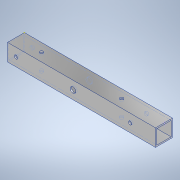
# Autodesk Inventor part: ロボットベース15x15_3
Saved by Autodesk Inventor 2020.3 (Build 243373000, 373)
## iProperties
Created: 2020-07-04
Part Number: ロボットベース15x15_3
Material: アルミニウム 6061
Document SubType Name: Modeling
Designer: totot
Density: 2.7 g/cm^3
Appearance: アルミニウム - フラット
Mass: 20.4359 g
Surface Area: 128.754 cm^2
Volume: 7.56886 cm^3
Author: totot
Autodesk Inventor part; units mm, degrees
ref_plane "YZ Plane" through (0, 0, 0) normal (1, 0, 0) x (0, 1, 0)
ref_plane "XZ Plane" through (0, 0, 0) normal (0, 1, 0) x (-1, 0, 0)
ref_plane "XY Plane" through (0, 0, 0) normal (0, 0, 1) x (1, 0, 0)
sketch "スケッチ1" plane through (0, 0, 0) normal (1, 0, 0) x (0, 1, 0)
  line L0 (0, 0) -> (-15, 0)
  line L1 (-15, 0) -> (-15, 15)
  line L2 (-15, 15) -> (0, 15)
  line L3 (0, 15) -> (0, 0)
  line L4 (-1.2, 13.8) -> (-13.8, 13.8)
  line L5 (-13.8, 13.8) -> (-13.8, 1.2)
  line L6 (-13.8, 1.2) -> (-1.2, 1.2)
  line L7 (-1.2, 1.2) -> (-1.2, 13.8)
  dimension "d0" = 15
  dimension "d1" = 15
  dimension "d2" = 1.2
  dimension "d3" = 1.2
  dimension "d4" = 1.2
  dimension "d5" = 1.2
  constraints: 16 end point, 4 parallel, 2 horizontal, 2 perpendicular
  measures "d0" distance of L1.end L2.end
  measures "d1" distance of L0.end L1.end
  measures "d2" distance between parallel lines of L2 L4
  measures "d3" distance between parallel lines of L7 L3
  measures "d4" distance between parallel lines of L1 L5
  measures "d5" distance between parallel lines of L0 L6
extrude "押し出し1" add sketch "スケッチ1" along normal blind 116
sketch "スケッチ2" plane through (0, -15, 15) normal (0, 0, 1) x (1, 0, 0)
  line L0 (0, 15) -> (116, 15) projected
  line L1 (0, 15) -> (0, 0) projected
  line L2 (116, 15) -> (116, 0) projected
  point P0 (7.5, 7.5)
  point P1 (108.5, 7.5)
  dimension "d8" = 7.5
  dimension "d9" = 7.5
  dimension "d10" = 7.5
  dimension "d11" = 7.5
  measures "d8" distance from line of L0 point (7.5, 7.5)
  measures "d9" distance from line of point (108.5, 7.5) L0
  measures "d10" distance from line of point (7.5, 7.5) L1
  measures "d11" distance from line of point (108.5, 7.5) L2
hole "穴1" at (7.5, -7.5, 15) at (108.5, -7.5, 15) direction (0, 0, -1) diameter 3 end through all
sketch "スケッチ3" plane through (0, -15, 0) normal (0, 0, -1) x (-1, 0, 0)
  circle A0 centre (-7.5, 7.5) radius 1.5 projected
  line L0 (0, 0) -> (-116, 0) projected
  point P0 (0, 15)
  point P1 (-58, 7.5)
  dimension "d19" = 50.5
  dimension "d20" = 7.5
  measures "d19" distance of point (-58, 7.5) A0.centre
  measures "d20" distance from line of point (-58, 7.5) L0
hole "穴2" at (58, -7.5, 0) direction (0, 0, 1) diameter 5 end through all
sketch "スケッチ4" plane through (0, -15, 0) normal (0, -1, 0) x (1, 0, 0)
  line L0 (0, 15) -> (0, 0) projected
  line L1 (0, 0) -> (116, 0) projected
  line L2 (116, 15) -> (116, 0) projected
  point P0 (22.5, 7.5)
  point P1 (93.5, 7.5)
  dimension "d28" = 22.5
  dimension "d29" = 7.5
  dimension "d30" = 7.5
  dimension "d31" = 22.5
  measures "d28" distance from line of point (22.5, 7.5) L0
  measures "d29" distance from line of point (22.5, 7.5) L1
  measures "d30" distance from line of L1 point (93.5, 7.5)
  measures "d31" distance from line of point (93.5, 7.5) L2
hole "穴3" at (22.5, -15, 7.5) at (93.5, -15, 7.5) direction (0, 1, 0) diameter 3 end through all
sketch "スケッチ5" plane through (116, 0, 0) normal (1, 0, 0) x (0, 0, -1)
  line L0 (0, 0) -> (-15, 0)
  line L1 (-15, 0) -> (-15, -15)
  line L2 (-15, -15) -> (0, -15)
  line L3 (0, -15) -> (0, 0)
  line L4 (-13.8, -1.2) -> (-1.2, -1.2) projected
  line L5 (-1.2, -1.2) -> (-13.8, -1.2)
  line L6 (-13.8, -1.2) -> (-13.8, -13.8)
  line L7 (-13.8, -13.8) -> (-1.2, -13.8)
  line L8 (-1.2, -13.8) -> (-1.2, -1.2)
  dimension "d39" = 15
  dimension "d40" = 15
  constraints: 16 end point, 4 parallel, 2 horizontal, 2 perpendicular
  measures "d39" distance of L2.end L1.end
  measures "d40" distance of L1.end L0.end
extrude "押し出し2" add sketch "スケッチ5" along normal blind 99
sketch "スケッチ6" plane through (0, -15, 0) normal (0, 0, -1) x (-1, 0, 0)
  line L0 (-215, 0) -> (-215, 15) projected
  line L1 (0, 15) -> (-215, 15) projected
  point P0 (-207.5, 7.5)
  dimension "d43" = 7.5
  dimension "d44" = 7.5
  measures "d43" distance from line of L0 point (-207.5, 7.5)
  measures "d44" distance from line of L1 point (-207.5, 7.5)
hole "穴4" at (207.5, -7.5, 0) direction (0, 0, 1) diameter 3 end through all
sketch "スケッチ7" plane through (0, 0, 15) normal (0, 1, 0) x (1, 0, 0)
  line L0 (0, 15) -> (215, 15) projected
  line L1 (215, 15) -> (215, 0) projected
  point P0 (192.5, 7.5)
  dimension "d52" = 7.5
  dimension "d53" = 22.5
  measures "d52" distance from line of L0 point (192.5, 7.5)
  measures "d53" distance from line of L1 point (192.5, 7.5)
hole "穴5" at (192.5, 0, 7.5) direction (0, -1, 0) diameter 3 end through all
sketch "スケッチ8" plane through (0, -15, 0) normal (0, 0, -1) x (-1, 0, 0)
  circle A0 centre (-108.5, 7.5) radius 1.5 projected
  line L0 (0, 0) -> (-215, 0) projected
  line L1 (-215, 0) -> (-215, 15) projected
  point P0 (0, 15)
  point P1 (-131, 7.5)
  point P2 (-177.5, 7.5)
  dimension "d61" = 22.5
  dimension "d62" = 7.5
  dimension "d63" = 7.5
  dimension "d64" = 37.5
  measures "d61" distance of point (-131, 7.5) A0.centre
  measures "d62" distance from line of point (-131, 7.5) L0
  measures "d63" distance from line of L0 point (-177.5, 7.5)
  measures "d64" distance from line of L1 point (-177.5, 7.5)
hole "穴6" at (131, -7.5, 0) at (177.5, -7.5, 0) direction (0, 0, 1) diameter 3 end through all
equation "\"d3\" = d2"
equation "\"d4\" = d2"
equation "\"d5\" = d3"
equation "\"d9\" = d8"
equation "\"d10\" = d8"
equation "\"d11\" = d9"
equation "\"d30\" = d29"
equation "\"d31\" = d28"
equation "\"d63\" = d62"
